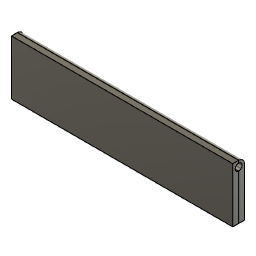
front+bottom+cover (Autodesk Fusion 360 design; units mm, degrees)
Autodesk Fusion 360 part; units mm, degrees
sketch "Sketch1" plane through (0, 0, 0) normal (0, 0, 1) x (1, 0, 0)
  line L0 (0, 0) -> (175, 0)
  line L1 (175, 0) -> (175, 46.35)
  line L2 (175, 46.35) -> (0, 46.35)
  line L3 (0, 46.35) -> (0, 0)
  dimension "d1" = 175
  dimension "d2" = 46.35
  constraint horizontal L0
  constraint vertical L1
  constraint horizontal L2
  constraint vertical L3
  constraint coincident L0.start L3.end
  measures "d1" distance of L0.start L0.end
  measures "d2" distance of L0.start L2.end
extrude "Extrude1" add sketch "Sketch1" along normal blind 8 makes body 1
extrude "Extrude2" add 1 faces at (58.3333, 30.9, 8) along direction (0, 0, 1) blind 2 on bodies 1 bodies 1
sketch "Sketch2" plane through (175, 0, 0) normal (1, 0, 0) x (0, 0, -1)
  line L0 (0, 0) -> (0, 46.35)
  line L1 (0, 46.35) -> (-10, 46.35)
  line L2 (-10, 46.35) -> (-10, 0)
  line L3 (-10, 0) -> (0, 0)
  circle A0 centre (-5, 41) radius 3
  dimension "d7" = 6
  measures "d7" diameter of A0
extrude "Extrude3" cut sketch "Sketch2" against normal blind 10 contours A0 bodies 1
sketch "Sketch3" plane through (0, 0, 0) normal (1, 0, 0) x (0, 0, -1)
sketch "Sketch4" plane through (0, 0, 0) normal (-1, 0, 0) x (0, 0, 1)
  line L0 (0, 46.35) -> (0, 0)
  line L1 (0, 0) -> (10, 0)
  line L2 (10, 0) -> (10, 46.35)
  line L3 (10, 46.35) -> (0, 46.35)
  circle A0 centre (5, 41) radius 3
  dimension "d10" = 6
  dimension "d11" = 5.35
  measures "d10" diameter of A0
  measures "d11" distance of L3 A0.centre
extrude "Extrude4" cut sketch "Sketch4" against normal blind 10 contours A0 bodies 1
sketch "Sketch5" plane through (0, 0, 0) normal (0, 0, 1) x (1, 0, 0)
sketch "Sketch6" plane through (0, 0, 0) normal (-1, 0, 0) x (0, 0, 1)
  circle A0 centre (5, 41) radius 3
  line L0 (0, 46.35) -> (0, 0)
  line L1 (0, 0) -> (10, 0)
  line L2 (10, 0) -> (10, 46.35)
  line L3 (10, 46.35) -> (0, 46.35)
  arc A1 (5, 46) -> (0, 41) centre (5, 41) ccw
  line L4 (5, 46) -> (10, 46)
  line L5 (0, 41) -> (0, 46.35)
  line L6 (10, 46.35) -> (0, 46.35)
  line L7 (10, 46.35) -> (10, 46)
  constraint concentric A0 A1
  constraint tangent L0 A1
  constraint coincident L0 A1.end
  constraint coincident L2 L4.end
  constraint tangent A1 L4
  constraint perpendicular L2 L4
  constraint coincident L0.start L3.end
  constraint coincident L2.end L3.start
extrude "Extrude5" cut sketch "Sketch6" against normal through all contours L0 L2 L3 A1 L4 L5 L6 L7 bodies 1
ref_plane "WorkPlane1" through (87.5, 23.175, 5) normal (0, 0, -1) x (-1, 0, 0)
extrude "Extrude6" add 2 faces at (58.3333, 0, 3.3333) (58.3333, 0, 3.3333) along direction (0, -1, 0) blind 0.381 on bodies 1 bodies 1
extrude "Extrude7" add 1 faces at (175, 12.4155, 4.9253) along direction (1, 0, 0) blind 12.7 on bodies 1 bodies 1
split "Split3" by plane through (87.5, 23.175, 5) normal (0, 0, -1) bodies 1 makes body 2 at (125.1333, 13.4127, 0)
